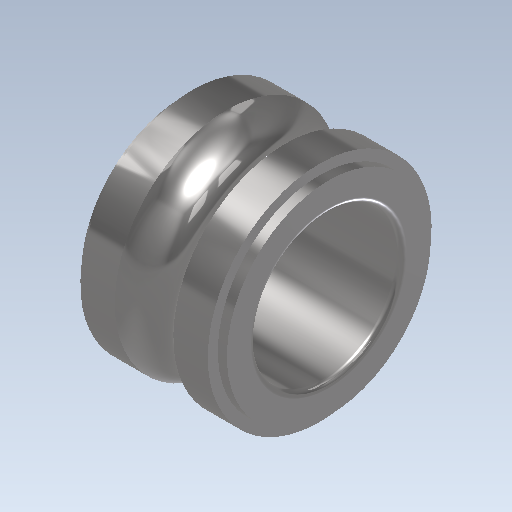
# Autodesk Inventor part: F694ZZ Inner Ring
Saved by Autodesk Inventor 2020.3 (Build 243373000, 373)
## iProperties
Created: 2018-10-12
Part Number: F694ZZ Inner Ring
Material: ステンレス鋼 440C
Catalog Web Link: www.cadenas.de
Description: shielded_type_zz_zzs_IR-
Vendor: NSK_RB
Document SubType Name: Modeling
Designer: psadmin
Manufacturer: NSK_RB
Mass: 0.451052 g
Surface Area: 1.60849 cm^2
Volume: 0.0582002 cm^3
Density: 7.75 g/cm^3
Appearance: 半つや出し
Category: PARTsolutions
Company: NSK_RB
PSOL_IDENT_0: {$CADENAS_DATA\23d-libs\nsk_rb\roller_bearings\deep_groove_bb\exstra_small_miniatur_bb\metric_design
PSOL_IDENT_1: _with_flange\shielded_type_zz_zzs_ir_1.prj},192 {VTYP=3D},{NB=F694ZZ Inner Ring},{LINA=F694ZZ Inner
PSOL_IDENT_2: Ring},{NN=shielded_type_zz_zzs_IR},{DATE=18.07.2018 08:51:05},{GEOMDATE=04.01.2008 00:00:00},{VERSIO
PSOL_IDENT_3: N=},{LINEID=250},{WBVAR=},{WBNUMERIC=}  {NB=F694ZZ Inner Ring},{LINA=F694ZZ Inner Ring},{KT=DUMMY},{
PSOL_IDENT_4: IDNR=},{STAN=},{ORDER=F694ZZ},{SD=4.0},{X=4.0},{D=11},{DD=11},{DD1=0.0},{D2=12.5},{DD2=12.5},{B=0.0}
PSOL_IDENT_5: ,{B1=4.0},{CC1=0.0},{C2=1.0},{CC2=1.0},{R=0.00},{R1=0.15},{DI1=6.15},{DI2=5.60},{SDE1=8.95},{SDE2=9.
PSOL_IDENT_6: 85},{CR1=960},{COR1=345},{CR2=98},{COR2=35.0},{LG=48000},{LO=56000},{DA=0.0},{DB=5.6},{RA=0.00},{RB=
PSOL_IDENT_7: 0.15},{MASS=1.96},{SC=1},{N=8}
NN: shielded_type_zz_zzs_IR
NB: F694ZZ Inner Ring
NBSYN: $ORDER. Inner Ring
LINA: F694ZZ Inner Ring
ORDER: F694ZZ
SD: 4
X: 4
D: 11
DD: 11
DD1: 0
D2: 0
DD2: 12.5
B: 0
B1: 4
CC1: 0
C2: 1
CC2: 1
R: 0
R1: 0.15
DI1: 6.15
DI2: 5.6
SDE1: 8.95
SDE2: 9.85
CR1: 960
COR1: 345
CR2: 98
COR2: 35
LG: 48000
LO: 56000
DA: 0
DB: 5.6
RA: 0
RB: 0.15
MASS: 1.96
SC: 1
SUPPLIER: NSK_RB
ARTICLENO: F694ZZ Inner Ring
BOMINFO: F694ZZ Inner Ring
CREATOR: CADENAS GmbH
d1: 0.000 mm
Title: F694ZZ Inner Ring
Author: Cadenas PARTsolutions
Autodesk Inventor part; units mm, degrees
sketch "Sketch_2" plane through (0, 0, 0) normal (0, 0, 1) x (1, 0, 0)
  line L0 (4, 0) -> (0, 0)
  arc A0 (0, 2.15) -> (0.15, 2) centre (0.15, 2.15) ccw
  line L1 (0.15, 2) -> (3.85, 2)
  arc A1 (3.85, 2) -> (4, 2.15) centre (3.85, 2.15) ccw
  line L2 (4, 2.15) -> (4, 2.8)
  line L3 (4, 2.8) -> (3.75, 2.8)
  line L4 (3.75, 2.8) -> (3.75, 3.075)
  line L5 (3.75, 3.075) -> (2.8043, 3.075)
  arc A2 (1.1957, 3.075) -> (2.8043, 3.075) centre (2, 3.75) ccw
  line L6 (1.1957, 3.075) -> (0.25, 3.075)
  line L7 (0.25, 3.075) -> (0.25, 2.8)
  line L8 (0.25, 2.8) -> (0, 2.8)
  line L9 (0, 2.8) -> (0, 2.15)
  constraints: 20 end point, 6 point on circle, 3 centre point
revolve "Revolution1" add sketch "Sketch_2" angle 360 about axis through (4, 0, 0) along (1, 0, 0)
ref_plane "ip_st_1_1_XY" through (2, 3.75, 0) normal (1, 0, 0) x (0, 0, -1)
ref_plane "ip_st_1_1_YZ" through (2, 3.75, 0) normal (0, 0, -1) x (0, 1, 0)
ref_plane "ip_st_1_1_ZX" through (2, 3.75, 0) normal (0, 1, 0) x (1, 0, 0)
ref_plane "ip_st_1_2_XY" through (2, 2.6517, 2.6517) normal (1, 0, 0) x (0, 0, -1)
ref_plane "ip_st_1_2_YZ" through (2, 2.6517, 2.6517) normal (0, 0, -1) x (0, 1, 0)
ref_plane "ip_st_1_2_ZX" through (2, 2.6517, 2.6517) normal (0, 1, 0) x (1, 0, 0)
ref_plane "ip_st_1_3_XY" through (2, 0, 3.75) normal (1, 0, 0) x (0, 0, -1)
ref_plane "ip_st_1_3_YZ" through (2, 0, 3.75) normal (0, 0, -1) x (0, 1, 0)
ref_plane "ip_st_1_3_ZX" through (2, 0, 3.75) normal (0, 1, 0) x (1, 0, 0)
ref_plane "ip_st_1_4_XY" through (2, -2.6517, 2.6517) normal (1, 0, 0) x (0, 0, -1)
ref_plane "ip_st_1_4_YZ" through (2, -2.6517, 2.6517) normal (0, 0, -1) x (0, 1, 0)
ref_plane "ip_st_1_4_ZX" through (2, -2.6517, 2.6517) normal (0, 1, 0) x (1, 0, 0)
ref_plane "ip_st_1_5_XY" through (2, -3.75, 0) normal (1, 0, 0) x (0, 0, -1)
ref_plane "ip_st_1_5_YZ" through (2, -3.75, 0) normal (0, 0, -1) x (0, 1, 0)
ref_plane "ip_st_1_5_ZX" through (2, -3.75, 0) normal (0, 1, 0) x (1, 0, 0)
ref_plane "ip_st_1_6_XY" through (2, -2.6517, -2.6517) normal (1, 0, 0) x (0, 0, -1)
ref_plane "ip_st_1_6_YZ" through (2, -2.6517, -2.6517) normal (0, 0, -1) x (0, 1, 0)
ref_plane "ip_st_1_6_ZX" through (2, -2.6517, -2.6517) normal (0, 1, 0) x (1, 0, 0)
ref_plane "ip_st_1_7_XY" through (2, 0, -3.75) normal (1, 0, 0) x (0, 0, -1)
ref_plane "ip_st_1_7_YZ" through (2, 0, -3.75) normal (0, 0, -1) x (0, 1, 0)
ref_plane "ip_st_1_7_ZX" through (2, 0, -3.75) normal (0, 1, 0) x (1, 0, 0)
ref_plane "ip_st_1_8_XY" through (2, 2.6517, -2.6517) normal (1, 0, 0) x (0, 0, -1)
ref_plane "ip_st_1_8_YZ" through (2, 2.6517, -2.6517) normal (0, 0, -1) x (0, 1, 0)
ref_plane "ip_st_1_8_ZX" through (2, 2.6517, -2.6517) normal (0, 1, 0) x (1, 0, 0)
ref_plane "ip_st_1a_XY" through (0, 0, 0) normal (1, 0, 0) x (0, 0, -1)
ref_plane "ip_st_1a_YZ" through (0, 0, 0) normal (0, 0, -1) x (0, 1, 0)
ref_plane "ip_st_1a_ZX" through (0, 0, 0) normal (0, 1, 0) x (1, 0, 0)
ref_plane "ip_st_2a_XY" through (0.25, 0, 0) normal (1, 0, 0) x (0, 0, -1)
ref_plane "ip_st_2a_YZ" through (0.25, 0, 0) normal (0, 0, -1) x (0, 1, 0)
ref_plane "ip_st_2a_ZX" through (0.25, 0, 0) normal (0, 1, 0) x (1, 0, 0)
body "Solid1"
